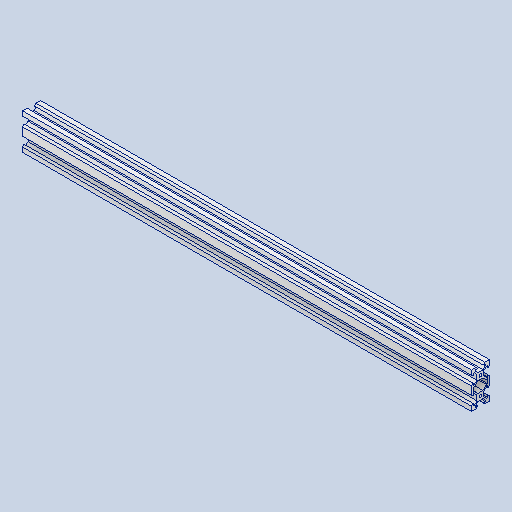
# Autodesk Inventor part: Riel Banda
Saved by Autodesk Inventor 2025 (Build 290162000, 162)
## iProperties
Created: 2026-09-20
Part Number: Riel Banda
Material: Aluminio 6061
Document SubType Name: Modeling
Designer: ASUS
Density: 2.7 g/cm^3
Appearance: Aluminio - Plano
Author: ASUS
Autodesk Inventor part; units mm, degrees
ref_plane "YZ Plane" through (0, 0, 0) normal (1, 0, 0) x (0, 1, 0)
ref_plane "XZ Plane" through (0, 0, 0) normal (0, 1, 0) x (-1, 0, 0)
ref_plane "XY Plane" through (0, 0, 0) normal (0, 0, 1) x (1, 0, 0)
sketch "Boceto1" plane through (0, 0, 0) normal (1, 0, 0) x (0, 1, 0)
  line L0 (20, 10) -> (20, 4.9)
  line L1 (20, -10) -> (20, -4.9)
  line L2 (20, -4.9) -> (18.2, -3.1)
  line L3 (18.2, -3.1) -> (18.2, -5.461)
  line L4 (20, 4.9) -> (18.2, 3.1)
  line L5 (20, 4.9) -> (22.5456, 4.9) construction
  line L6 (18.2, 3.1) -> (18.2, 5.5)
  line L7 (20, -10) -> (14.9, -10)
  line L8 (20, 10) -> (14.9, 10)
  line L9 (14.9, 10) -> (13.1, 8.2)
  line L10 (15.5, 8.2) -> (13.1, 8.2)
  line L11 (-20, 10) -> (-20, 4.9)
  line L12 (-20, 10) -> (-14.9, 10)
  line L13 (-14.9, 10) -> (-13.1, 8.2)
  line L14 (-20, 10) -> (-18.2, 10)
  line L15 (-18.2, 3.1) -> (-20, 4.9)
  line L16 (-20, -10) -> (-14.9, -10)
  line L17 (-20, -10) -> (-20, -4.9)
  line L18 (-14.9, -10) -> (-13.1, -10) construction
  line L19 (-20, -4.9) -> (-18.2, -3.1)
  line L20 (-18.2, -3.1) -> (-18.2, -5.5)
  line L21 (-13.1, 8.2) -> (-15.4583, 8.2)
  line L22 (-18.2, 3.1) -> (-18.2, 5.5)
  circle A0 centre (10, -0.0059) radius 1.7
  circle A1 centre (-10, -0.0177) radius 1.7
  line L23 (15.5, 8.2) -> (15.5, 6.561)
  line L24 (18.2, 5.5) -> (16.561, 5.5)
  line L25 (14.9, -10) -> (13.1, -8.2)
  line L26 (13.1, -8.2) -> (15.5, -8.2)
  line L27 (18.2, -5.461) -> (16.6, -5.461)
  line L28 (15.5, -8.2) -> (15.5, -6.561)
  line L29 (-15.4583, 8.2) -> (-15.4583, 6.5999)
  line L30 (-18.2, 5.5) -> (-16.561, 5.5)
  line L31 (-18.2, -5.5) -> (-16.561, -5.5)
  line L32 (-14.9, -10) -> (-13.1, -8.2)
  line L33 (-13.1, -8.2) -> (-15.4611, -8.2)
  line L34 (-15.4611, -8.2) -> (-15.4611, -6.6001)
  line L35 (16.561, 5.5) -> (13.9, 2.7941)
  line L36 (15.5, 6.561) -> (12.8, 3.8941)
  line L37 (16.6, -5.461) -> (13.9, -2.8059)
  line L38 (15.5, -6.561) -> (12.8, -3.9059)
  line L39 (-15.4611, -6.6001) -> (-12.8, -3.9177)
  line L40 (-16.561, -5.5) -> (-13.9, -2.8177)
  line L41 (-15.4583, 6.5999) -> (-12.7974, 3.8823)
  line L42 (-16.561, 5.5) -> (-13.9, 2.7823)
  line L43 (4.5, -10) -> (-4.5, -10)
  line L44 (4.5, 10) -> (-4.5, 10)
  line L45 (4.5, 10) -> (6.4646, 8.241)
  line L46 (-4.5, 10) -> (-6.2418, 8.2)
  line L47 (6.4646, 8.241) -> (4.0646, 8.241)
  line L48 (-6.2418, 8.2) -> (-3.8392, 8.2)
  line L49 (-3.8392, 8.2) -> (-3.8392, 7.2)
  line L50 (-4.5, -10) -> (-6.2418, -8.2)
  line L51 (-6.2418, -8.2) -> (-3.8418, -8.2)
  line L52 (4.5, -10) -> (6.4219, -8.2)
  line L53 (6.4219, -8.2) -> (4.0173, -8.2)
  line L54 (-3.8392, 7.2) -> (-7.1974, 3.8823)
  line L55 (-2.3392, 8.1975) -> (2.5289, 8.1975)
  line L56 (-2.3392, 8.1975) -> (-2.3392, 6.6975)
  line L57 (-2.3392, 6.6975) -> (-6.1, 2.7823)
  line L58 (4.0646, 8.241) -> (4.0646, 7.241)
  line L59 (4.0646, 7.241) -> (7.1266, 3.8941)
  line L60 (2.5289, 8.1975) -> (2.5289, 6.6975)
  line L61 (2.5289, 6.6975) -> (6.1, 2.7941)
  line L62 (4.0173, -8.2) -> (4.0173, -7.1955)
  line L63 (4.0173, -7.1955) -> (7.2, -3.9059)
  line L64 (2.5289, -8.1957) -> (-2.3348, -8.1957)
  line L65 (2.5289, -8.1957) -> (2.5289, -6.6957)
  line L66 (2.5289, -6.6957) -> (6.1, -2.8059)
  line L67 (-3.8418, -8.2) -> (-3.8418, -7.2)
  line L68 (-3.8418, -7.2) -> (-7.2, -3.9177)
  line L69 (-2.3348, -8.1957) -> (-2.3348, -6.6957)
  line L70 (-2.3348, -6.6957) -> (-6.1, -2.8177)
  line L71 (12.8, -3.9059) -> (7.2, -3.9059)
  line L72 (6.1, -2.8059) -> (6.1, 2.7941)
  line L73 (7.1266, 3.8941) -> (12.8, 3.8941)
  line L74 (13.9, 2.7941) -> (13.9, -2.8059)
  line L75 (-7.1974, 3.8823) -> (-12.7974, 3.8823)
  line L76 (-6.1, 2.7823) -> (-6.1, -2.8177)
  line L77 (-7.2, -3.9177) -> (-12.8, -3.9177)
  line L78 (-13.9, -2.8177) -> (-13.9, 2.7823)
  point P0 (0, 0)
  point P1 (0, -10)
  point P2 (20, 0)
  point P3 (-20, 0)
  dimension "d4" = 40
  dimension "d5" = 20
  dimension "d6" = 5.1
  dimension "d7" = 5.1
  dimension "d13" = 1.8
  dimension "d16" = 135
  dimension "d18" = 5.1
  dimension "d31" = 2.4
  dimension "d32" = 5.1
  dimension "d33" = 5.1
  dimension "d41" = 5.1
  dimension "d55" = 3.4
  dimension "d59" = 10
  dimension "d65" = 20
  dimension "d70" = 1.639
  dimension "d72" = 1.639
  dimension "d80" = 1.639
  dimension "d100" = 9
  dimension "d101" = 15.5
  dimension "d104" = 2.4
  dimension "d108" = 1
  dimension "d110" = 9
  dimension "d111" = 15.5
  dimension "d115" = 1.5
  dimension "d116" = 1.5
  dimension "d119" = 1.5
  dimension "d123" = 1.5
  dimension "d124" = 1
  dimension "d125" = 1.5
  dimension "d126" = 1.5
  dimension "d127" = 1.5
  constraints: 158 end point, 15 horizontal, 14 vertical, 8 perpendicular, 6 parallel, 2 centre point, 2 point on line, 1 equal length, 1 horizontal alignment, 1 vertical alignment
  measures "d4" distance of L1.start L16.start
  measures "d5" distance of L16.start L11.start
  measures "d6" distance of L0.start L0.end
  measures "d7" distance of L1.start L1.end
  measures "d13" horizontal distance of L1.end L2.end
  measures "d16" angle of L4 L5
  measures "d18" distance of L1.start L7.end
  measures "d31" distance of L10.start L9.end
  measures "d32" distance of L11.start L11.end
  measures "d33" distance of L11.start L12.end
  measures "d41" distance of L16.start L16.end
  measures "d55" diameter of A1
  measures "d59" distance of A0.centre point (20, 0)
  measures "d65" distance of A1.centre A0.centre
  measures "d70" distance of L6.end L24.end
  measures "d72" distance of L10.start L23.end
  measures "d80" distance of L22.end L30.end
  measures "d100" distance of L43.start L43.end
  measures "d101" distance of L43.start L1.start
  measures "d104" distance of L45.end L47.end
  measures "d108" distance of L48.end L49.end
  measures "d110" distance of L44.start L44.end
  measures "d111" distance of L44.start L0.start
  measures "d115" distance of L55.start L56.end
  measures "d116" angle of L57 L54
  measures "d119" distance of L55.end L60.end
  measures "d123" distance of L64.start L65.end
  measures "d124" distance of L51.end L67.end
  measures "d125" distance of L64.end L69.end
  measures "d126" angle of L68 L70
  measures "d127" angle of L66 L63
extrude "Extrusión1" add sketch "Boceto1" along normal blind 500
